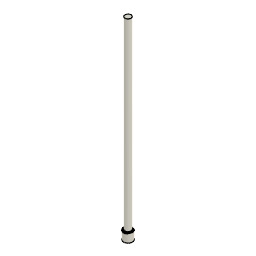
M3x5x4mm Heatset Bridge Cutter (Autodesk Fusion 360 design; units mm, degrees)
Autodesk Fusion 360 part; units mm, degrees
note: some values were not read from the file. Set by a fixed rule: which sketch regions a step uses.
sketch "Sketch1" plane through (0, 0, 0) normal (0, 0, 1) x (1, 0, 0)
  circle A0 centre (0, 0) radius 2.35
  dimension "d1" = 4.7
  constraint coincident A0.centre origin
  measures "d1" diameter of A0
extrude "Extrude1" add sketch "Sketch1" along normal blind 4.2
sketch "Sketch2" plane through (0, 0, 4.2) normal (0, 0, 1) x (-1, 0, 0)
  circle A0 centre (0, 0) radius 2.35
  circle A1 centre (0, 0) radius 1.6
  dimension "d4" = 3.2
  constraint coincident A0.centre A1.centre
  measures "d4" diameter of A1
extrude "Extrude2" add sketch "Sketch2" along normal blind 100 from surface at -4.2 contours A1
sketch "Sketch3" plane through (0, 0, 4.2) normal (0, 0, 1) x (-1, 0, 0)
  circle A0 centre (0, 0) radius 1.6
  circle A1 centre (0, 0) radius 2.35
  line L0 (1.7212, -1.6) -> (-1.7212, -1.6)
  line L1 (1.7212, 1.6) -> (-1.7212, 1.6)
  constraint coincident A1 L0.start
  constraint coincident A1 L0.end
  constraint horizontal L0
  constraint tangent A0 L0
  constraint coincident A1 L1.start
  constraint coincident A1 L1.end
  constraint horizontal L1
  constraint tangent A0 L1
extrude "Extrude3" add sketch "Sketch3" along normal blind 0.2 contours A0 A1 L0 L1 | A0 A1 L0 L1
sketch "Sketch4" plane through (0, 0, 4.4) normal (0, 0, 1) x (-1, 0, 0)
  arc A0 (1.7212, -1.6) -> (1.7212, 1.6) centre (0, 0) ccw
  line L0 (1.7212, 1.6) -> (0, 1.6)
  arc A1 (0, -1.6) -> (0, 1.6) centre (0, 0) ccw
  line L1 (0, -1.6) -> (1.7212, -1.6)
  line L2 (0, 1.6) -> (-1.7212, 1.6)
  arc A2 (-1.7212, 1.6) -> (-1.7212, -1.6) centre (0, 0) ccw
  line L3 (-1.7212, -1.6) -> (0, -1.6)
  arc A3 (0, 1.6) -> (0, -1.6) centre (0, 0) ccw
  line L4 (1.6, -1.6) -> (1.6, 1.6)
  line L5 (-1.6, 1.6) -> (-1.6, -1.6)
  constraint coincident L1 L4.start
  constraint coincident L0 L4.end
  constraint perpendicular L0 L4
  constraint tangent A1 L4
  constraint coincident L2 L5.start
  constraint coincident L3 L5.end
  constraint perpendicular L3 L5
  constraint tangent A3 L5
extrude "Extrude4" add sketch "Sketch4" along normal blind 0.2 contours A1 L1 L4 | L0 A1 L4 | L3 A3 L5 | L2 A3 L5
